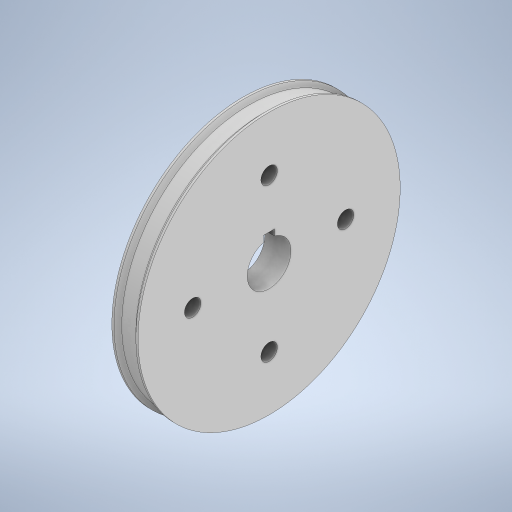
# Autodesk Inventor part: Polea clase #2
Saved by Autodesk Inventor 2024 (Build 280153000, 153)
## iProperties
Created: 2024-02-06
Part Number: Polea clase #2
Material: Genérico
Document SubType Name: Modeling
Designer: Adrian Montalvan
Density: 1 g/cm^3
Appearance: Valor por defecto
Author: Adrian Montalvan
Autodesk Inventor part; units mm, degrees
ref_plane "YZ Plane" through (0, 0, 0) normal (1, 0, 0) x (0, 1, 0)
ref_plane "XZ Plane" through (0, 0, 0) normal (0, 1, 0) x (-1, 0, 0)
ref_plane "XY Plane" through (0, 0, 0) normal (0, 0, 1) x (1, 0, 0)
sketch "Boceto1" plane through (0, 0, 0) normal (0, 0, 1) x (1, 0, 0)
  line L0 (0, 0) -> (100, 0)
  line L1 (100, 0) -> (100, 500)
  line L2 (0, 500) -> (0, 0)
  line L3 (0, 500) -> (17.6777, 482.3223)
  line L4 (0, 500) -> (25, 500) construction
  line L5 (100, 500) -> (82.3223, 482.3223)
  line L6 (82.3223, 482.3223) -> (17.6777, 482.3223)
  line L7 (50, -100) -> (-150, -100)
  dimension "d1" = 500
  dimension "d2" = 25
  dimension "d3" = 45
  dimension "d4" = 25
  dimension "d6" = 200
  constraints: 16 end point, 4 horizontal, 1 equal length, 1 parallel, 1 perpendicular
  measures "d1" distance of L1.end L0.end
  measures "d2" distance of L2.start L3.end
  measures "d3" angle of L3 L4
  measures "d4" distance of L1.end L5.end
  measures "d6" distance of L7.start L7.end
revolve "Revolución1" add sketch "Boceto1" angle 360 about axis through (50, -100, 0) along (-1, 0, 0)
sketch "Boceto2" plane through (100, -100, 0) normal (1, 0, 0) x (0, 0, -1)
  circle A0 centre (0, 0) radius 600 projected
  circle A1 centre (0, 350) radius 37.5
  circle A2 centre (-350, 0) radius 37.5
  circle A3 centre (0, -350) radius 37.5
  circle A4 centre (350, 0) radius 37.5
  point P0 (0, 100)
  dimension "d11" = 360
  constraints: 4 centre point, 1 coincident, 9 other
extrude "Extrusión1" cut sketch "Boceto2" against normal blind 100 contours A1 | A2 | A3 | A4
thicken "Engrosado1" operation add thickness 10 both sides no extend neighbours no toward (1, 0, 0) faces at (100, -364.9419, 262.9039)
thicken "Engrosado2" operation add thickness 10 both sides no extend neighbours no toward (-1, 0, 0) faces at (0, -364.9419, 262.9039)
sketch "Boceto3" plane through (110, -100, 0) normal (1, 0, 0) x (0, 0, -1)
  line L0 (-25, 125) -> (25, 125)
  line L1 (25, 125) -> (25, 96.8246)
  line L2 (-25, 96.8246) -> (-25, 125)
  line L3 (-25, 125) -> (25, 75) construction
  line L4 (25, 125) -> (-25, 75) construction
  arc A0 (25, 96.8246) -> (-25, 96.8246) centre (0, 0) ccw
  point P0 (0, 100)
  constraints: 10 end point, 2 midpoint, 2 point on circle, 1 centre point, 1 horizontal, 1 parallel, 1 perpendicular
extrude "Extrusión2" cut sketch "Boceto3" against normal blind 120
